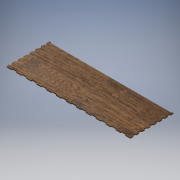
# Autodesk Inventor part: tavolaBase
Saved by Autodesk Inventor 2018.3 (Build 223284000, 284)
## iProperties
Created: 2019-03-04
Part Number: tavolaBase
Material: Generico
Document SubType Name: Modeling
Designer: AlfyPc
Density: 1 g/cm^3
Appearance: Frassino bianco - Giava
Author: AlfyPc
Autodesk Inventor part; units mm, degrees
(part 1 of 2)
ref_plane "YZ Plane" through (0, 0, 0) normal (1, 0, 0) x (0, 1, 0)
ref_plane "XZ Plane" through (0, 0, 0) normal (0, 1, 0) x (-1, 0, 0)
ref_plane "XY Plane" through (0, 0, 0) normal (0, 0, 1) x (1, 0, 0)
sketch "Schizzo1" plane through (0, 0, 0) normal (0, 0, 1) x (1, 0, 0)
  line L0 (233.5, -78.5) -> (-233.5, -78.5)
  line L1 (-233.5, -78.5) -> (-233.5, 78.5)
  line L2 (-233.5, 78.5) -> (233.5, 78.5)
  line L3 (233.5, 78.5) -> (233.5, -78.5)
  line L4 (233.5, -78.5) -> (-233.5, 78.5) construction
  line L5 (-233.5, -78.5) -> (233.5, 78.5) construction
  point P0 (0, 0)
  dimension "d0" = 467
  dimension "d1" = 157
  constraints: 12 end point, 2 midpoint, 2 parallel, 1 horizontal, 1 perpendicular
  measures "d0" distance of L0.start L0.end
  measures "d1" distance of L0.end L1.end
extrude "Estrusione1" add sketch "Schizzo1" against normal blind 4
sketch "Schizzo3" plane through (0, 0, 0) normal (0, 0, 1) x (1, 0, 0)
  line L0 (233.5, -78.5) -> (-233.5, -78.5) projected
  line L1 (233.5, 78.5) -> (233.5, -78.5) projected
  line L2 (-233.5, 78.5) -> (233.5, 78.5) projected
  line L3 (-233.5, -78.5) -> (-233.5, 78.5) projected
  line L4 (-237.5, -82.5) -> (237.5, -82.5) construction
  line L5 (237.5, -82.5) -> (237.5, 82.5) construction
  line L6 (237.5, 82.5) -> (-237.5, 82.5) construction
  line L7 (-237.5, 82.5) -> (-237.5, -82.5) construction
  line L8 (237.5, -82.5) -> (218.5, -82.5)
  line L9 (218.5, -82.5) -> (218.5, -78.5)
  line L10 (218.5, -78.5) -> (237.5, -78.5)
  line L11 (237.5, -78.5) -> (237.5, -82.5)
  line L12 (237.5, 82.5) -> (218.5, 82.5)
  line L13 (218.5, 82.5) -> (218.5, 78.5)
  line L14 (218.5, 78.5) -> (237.5, 78.5)
  line L15 (237.5, 78.5) -> (237.5, 82.5)
  line L16 (237.5, -82.5) -> (233.5, -82.5)
  line L17 (233.5, -82.5) -> (233.5, -71.5)
  line L18 (233.5, -71.5) -> (237.5, -71.5)
  line L19 (237.5, -71.5) -> (237.5, -82.5)
  line L20 (-237.5, -82.5) -> (-233.5, -82.5)
  line L21 (-233.5, -82.5) -> (-233.5, -71.5)
  line L22 (-233.5, -71.5) -> (-237.5, -71.5)
  line L23 (-237.5, -71.5) -> (-237.5, -82.5)
  line L24 (218.5, -78.5) -> (218.5, -82.5)
  line L25 (218.5, -82.5) -> (214.5, -82.5)
  line L26 (199.5, -82.5) -> (199.5, -78.5)
  line L27 (199.5, -78.5) -> (218.5, -78.5)
  line L28 (218.5, -82.5) -> (199.5, -82.5)
  line L29 (199.5, 82.5) -> (199.5, 78.5)
  line L30 (199.5, 78.5) -> (218.5, 78.5)
  line L31 (218.5, 78.5) -> (218.5, 82.5)
  line L32 (218.5, 82.5) -> (199.5, 82.5)
  line L33 (199.5, -78.5) -> (199.5, -82.5)
  line L34 (199.5, -82.5) -> (195.5, -82.5)
  line L35 (180.5, -82.5) -> (180.5, -78.5)
  line L36 (180.5, -78.5) -> (199.5, -78.5)
  line L37 (199.5, -82.5) -> (180.5, -82.5)
  line L38 (180.5, 82.5) -> (180.5, 78.5)
  line L39 (180.5, 78.5) -> (199.5, 78.5)
  line L40 (199.5, 78.5) -> (199.5, 82.5)
  line L41 (199.5, 82.5) -> (180.5, 82.5)
  line L42 (180.5, -78.5) -> (180.5, -82.5)
  line L43 (180.5, -82.5) -> (176.5, -82.5)
  line L44 (161.5, -82.5) -> (161.5, -78.5)
  line L45 (161.5, -78.5) -> (180.5, -78.5)
  line L46 (180.5, -82.5) -> (161.5, -82.5)
  line L47 (161.5, 82.5) -> (161.5, 78.5)
  line L48 (161.5, 78.5) -> (180.5, 78.5)
  line L49 (180.5, 78.5) -> (180.5, 82.5)
  line L50 (180.5, 82.5) -> (161.5, 82.5)
  line L51 (161.5, -78.5) -> (161.5, -82.5)
  line L52 (161.5, -82.5) -> (157.5, -82.5)
  line L53 (142.5, -82.5) -> (142.5, -78.5)
  line L54 (142.5, -78.5) -> (161.5, -78.5)
  line L55 (161.5, -82.5) -> (142.5, -82.5)
  line L56 (142.5, 82.5) -> (142.5, 78.5)
  line L57 (142.5, 78.5) -> (161.5, 78.5)
  line L58 (161.5, 78.5) -> (161.5, 82.5)
  line L59 (161.5, 82.5) -> (142.5, 82.5)
  line L60 (142.5, -78.5) -> (142.5, -82.5)
  line L61 (142.5, -82.5) -> (138.5, -82.5)
  line L62 (123.5, -82.5) -> (123.5, -78.5)
  line L63 (123.5, -78.5) -> (142.5, -78.5)
  line L64 (142.5, -82.5) -> (123.5, -82.5)
  line L65 (123.5, 82.5) -> (123.5, 78.5)
  line L66 (123.5, 78.5) -> (142.5, 78.5)
  line L67 (142.5, 78.5) -> (142.5, 82.5)
  line L68 (142.5, 82.5) -> (123.5, 82.5)
  line L69 (123.5, -78.5) -> (123.5, -82.5)
  line L70 (123.5, -82.5) -> (119.5, -82.5)
  line L71 (104.5, -82.5) -> (104.5, -78.5)
  line L72 (104.5, -78.5) -> (123.5, -78.5)
  line L73 (123.5, -82.5) -> (104.5, -82.5)
  line L74 (104.5, 82.5) -> (104.5, 78.5)
  line L75 (104.5, 78.5) -> (123.5, 78.5)
  line L76 (123.5, 78.5) -> (123.5, 82.5)
  line L77 (123.5, 82.5) -> (104.5, 82.5)
  line L78 (104.5, -78.5) -> (104.5, -82.5)
  line L79 (104.5, -82.5) -> (100.5, -82.5)
  line L80 (85.5, -82.5) -> (85.5, -78.5)
  line L81 (85.5, -78.5) -> (104.5, -78.5)
  line L82 (104.5, -82.5) -> (85.5, -82.5)
  line L83 (85.5, 82.5) -> (85.5, 78.5)
  line L84 (85.5, 78.5) -> (104.5, 78.5)
  line L85 (104.5, 78.5) -> (104.5, 82.5)
  line L86 (104.5, 82.5) -> (85.5, 82.5)
  line L87 (85.5, -78.5) -> (85.5, -82.5)
  line L88 (85.5, -82.5) -> (81.5, -82.5)
  line L89 (66.5, -82.5) -> (66.5, -78.5)
  line L90 (66.5, -78.5) -> (85.5, -78.5)
  line L91 (85.5, -82.5) -> (66.5, -82.5)
  line L92 (66.5, 82.5) -> (66.5, 78.5)
  line L93 (66.5, 78.5) -> (85.5, 78.5)
  line L94 (85.5, 78.5) -> (85.5, 82.5)
  line L95 (85.5, 82.5) -> (66.5, 82.5)
  line L96 (66.5, -78.5) -> (66.5, -82.5)
  line L97 (66.5, -82.5) -> (62.5, -82.5)
  line L98 (47.5, -82.5) -> (47.5, -78.5)
  line L99 (47.5, -78.5) -> (66.5, -78.5)
  line L100 (66.5, -82.5) -> (47.5, -82.5)
  line L101 (47.5, 82.5) -> (47.5, 78.5)
  line L102 (47.5, 78.5) -> (66.5, 78.5)
  line L103 (66.5, 78.5) -> (66.5, 82.5)
  line L104 (66.5, 82.5) -> (47.5, 82.5)
  line L105 (47.5, -78.5) -> (47.5, -82.5)
  line L106 (47.5, -82.5) -> (43.5, -82.5)
  line L107 (28.5, -82.5) -> (28.5, -78.5)
  line L108 (28.5, -78.5) -> (47.5, -78.5)
  line L109 (47.5, -82.5) -> (28.5, -82.5)
  line L110 (28.5, 82.5) -> (28.5, 78.5)
  line L111 (28.5, 78.5) -> (47.5, 78.5)
  line L112 (47.5, 78.5) -> (47.5, 82.5)
  line L113 (47.5, 82.5) -> (28.5, 82.5)
  line L114 (28.5, -78.5) -> (28.5, -82.5)
  line L115 (28.5, -82.5) -> (24.5, -82.5)
  line L116 (9.5, -82.5) -> (9.5, -78.5)
  line L117 (9.5, -78.5) -> (28.5, -78.5)
  line L118 (28.5, -82.5) -> (9.5, -82.5)
  line L119 (9.5, 82.5) -> (9.5, 78.5)
  line L120 (9.5, 78.5) -> (28.5, 78.5)
  line L121 (28.5, 78.5) -> (28.5, 82.5)
  line L122 (28.5, 82.5) -> (9.5, 82.5)
  line L123 (9.5, -78.5) -> (9.5, -82.5)
  line L124 (9.5, -82.5) -> (5.5, -82.5)
  line L125 (-9.5, -82.5) -> (-9.5, -78.5)
  line L126 (-9.5, -78.5) -> (9.5, -78.5)
  line L127 (9.5, -82.5) -> (-9.5, -82.5)
  line L128 (-9.5, 82.5) -> (-9.5, 78.5)
  line L129 (-9.5, 78.5) -> (9.5, 78.5)
  line L130 (9.5, 78.5) -> (9.5, 82.5)
  line L131 (9.5, 82.5) -> (-9.5, 82.5)
  line L132 (-9.5, -78.5) -> (-9.5, -82.5)
  line L133 (-9.5, -82.5) -> (-13.5, -82.5)
  line L134 (-28.5, -82.5) -> (-28.5, -78.5)
  line L135 (-28.5, -78.5) -> (-9.5, -78.5)
  line L136 (-9.5, -82.5) -> (-28.5, -82.5)
  line L137 (-28.5, 82.5) -> (-28.5, 78.5)
  line L138 (-28.5, 78.5) -> (-9.5, 78.5)
  line L139 (-9.5, 78.5) -> (-9.5, 82.5)
  line L140 (-9.5, 82.5) -> (-28.5, 82.5)
  line L141 (-28.5, -78.5) -> (-28.5, -82.5)
  line L142 (-28.5, -82.5) -> (-32.5, -82.5)
  line L143 (-47.5, -82.5) -> (-47.5, -78.5)
  line L144 (-47.5, -78.5) -> (-28.5, -78.5)
  line L145 (-28.5, -82.5) -> (-47.5, -82.5)
  line L146 (-47.5, 82.5) -> (-47.5, 78.5)
  line L147 (-47.5, 78.5) -> (-28.5, 78.5)
  line L148 (-28.5, 78.5) -> (-28.5, 82.5)
  line L149 (-28.5, 82.5) -> (-47.5, 82.5)
  line L150 (-47.5, -78.5) -> (-47.5, -82.5)
  line L151 (-47.5, -82.5) -> (-51.5, -82.5)
  line L152 (-66.5, -82.5) -> (-66.5, -78.5)
  line L153 (-66.5, -78.5) -> (-47.5, -78.5)
  line L154 (-47.5, -82.5) -> (-66.5, -82.5)
  line L155 (-66.5, 82.5) -> (-66.5, 78.5)
  line L156 (-66.5, 78.5) -> (-47.5, 78.5)
  line L157 (-47.5, 78.5) -> (-47.5, 82.5)
  line L158 (-47.5, 82.5) -> (-66.5, 82.5)
  line L159 (-66.5, -78.5) -> (-66.5, -82.5)
  line L160 (-66.5, -82.5) -> (-70.5, -82.5)
  line L161 (-85.5, -82.5) -> (-85.5, -78.5)
  line L162 (-85.5, -78.5) -> (-66.5, -78.5)
  line L163 (-66.5, -82.5) -> (-85.5, -82.5)
  line L164 (-85.5, 82.5) -> (-85.5, 78.5)
  line L165 (-85.5, 78.5) -> (-66.5, 78.5)
  line L166 (-66.5, 78.5) -> (-66.5, 82.5)
  line L167 (-66.5, 82.5) -> (-85.5, 82.5)
  line L168 (-85.5, -78.5) -> (-85.5, -82.5)
  line L169 (-85.5, -82.5) -> (-89.5, -82.5)
  line L170 (-104.5, -82.5) -> (-104.5, -78.5)
  line L171 (-104.5, -78.5) -> (-85.5, -78.5)
  line L172 (-85.5, -82.5) -> (-104.5, -82.5)
  line L173 (-104.5, 82.5) -> (-104.5, 78.5)
  line L174 (-104.5, 78.5) -> (-85.5, 78.5)
  line L175 (-85.5, 78.5) -> (-85.5, 82.5)
  line L176 (-85.5, 82.5) -> (-104.5, 82.5)
  line L177 (-104.5, -78.5) -> (-104.5, -82.5)
  line L178 (-104.5, -82.5) -> (-108.5, -82.5)
  line L179 (-123.5, -82.5) -> (-123.5, -78.5)
  line L180 (-123.5, -78.5) -> (-104.5, -78.5)
  line L181 (-104.5, -82.5) -> (-123.5, -82.5)
  line L182 (-123.5, 82.5) -> (-123.5, 78.5)
  line L183 (-123.5, 78.5) -> (-104.5, 78.5)
  line L184 (-104.5, 78.5) -> (-104.5, 82.5)
  line L185 (-104.5, 82.5) -> (-123.5, 82.5)
  line L186 (-123.5, -78.5) -> (-123.5, -82.5)
  line L187 (-123.5, -82.5) -> (-127.5, -82.5)
  line L188 (-142.5, -82.5) -> (-142.5, -78.5)
  line L189 (-142.5, -78.5) -> (-123.5, -78.5)
  line L190 (-123.5, -82.5) -> (-142.5, -82.5)
  line L191 (-142.5, 82.5) -> (-142.5, 78.5)
  line L192 (-142.5, 78.5) -> (-123.5, 78.5)
  line L193 (-123.5, 78.5) -> (-123.5, 82.5)
  line L194 (-123.5, 82.5) -> (-142.5, 82.5)
  line L195 (-142.5, -78.5) -> (-142.5, -82.5)
  line L196 (-142.5, -82.5) -> (-146.5, -82.5)
  line L197 (-161.5, -82.5) -> (-161.5, -78.5)
  line L198 (-161.5, -78.5) -> (-142.5, -78.5)
  line L199 (-142.5, -82.5) -> (-161.5, -82.5)
  line L200 (-161.5, 82.5) -> (-161.5, 78.5)
  line L201 (-161.5, 78.5) -> (-142.5, 78.5)
  line L202 (-142.5, 78.5) -> (-142.5, 82.5)
  line L203 (-142.5, 82.5) -> (-161.5, 82.5)
  line L204 (-161.5, -78.5) -> (-161.5, -82.5)
  line L205 (-161.5, -82.5) -> (-165.5, -82.5)
  line L206 (-180.5, -82.5) -> (-180.5, -78.5)
  line L207 (-180.5, -78.5) -> (-161.5, -78.5)
  line L208 (-161.5, -82.5) -> (-180.5, -82.5)
  line L209 (-180.5, 82.5) -> (-180.5, 78.5)
  line L210 (-180.5, 78.5) -> (-161.5, 78.5)
  line L211 (-161.5, 78.5) -> (-161.5, 82.5)
  line L212 (-161.5, 82.5) -> (-180.5, 82.5)
  line L213 (-180.5, -78.5) -> (-180.5, -82.5)
  line L214 (-180.5, -82.5) -> (-184.5, -82.5)
  line L215 (-199.5, -82.5) -> (-199.5, -78.5)
  line L216 (-199.5, -78.5) -> (-180.5, -78.5)
  line L217 (-180.5, -82.5) -> (-199.5, -82.5)
  line L218 (-199.5, 82.5) -> (-199.5, 78.5)
  line L219 (-199.5, 78.5) -> (-180.5, 78.5)
  line L220 (-180.5, 78.5) -> (-180.5, 82.5)
  line L221 (-180.5, 82.5) -> (-199.5, 82.5)
  line L222 (-199.5, -78.5) -> (-199.5, -82.5)
  line L223 (-199.5, -82.5) -> (-203.5, -82.5)
  line L224 (-218.5, -82.5) -> (-218.5, -78.5)
  line L225 (-218.5, -78.5) -> (-199.5, -78.5)
  line L226 (-199.5, -82.5) -> (-218.5, -82.5)
  line L227 (-218.5, 82.5) -> (-218.5, 78.5)
  line L228 (-218.5, 78.5) -> (-199.5, 78.5)
  line L229 (-199.5, 78.5) -> (-199.5, 82.5)
  line L230 (-199.5, 82.5) -> (-218.5, 82.5)
  line L231 (-218.5, -78.5) -> (-218.5, -82.5)
  line L232 (-218.5, -82.5) -> (-222.5, -82.5)
  line L233 (-237.5, -82.5) -> (-237.5, -78.5)
  line L234 (-237.5, -78.5) -> (-218.5, -78.5)
  line L235 (-218.5, -82.5) -> (-237.5, -82.5)
  line L236 (-237.5, 82.5) -> (-237.5, 78.5)
  line L237 (-237.5, 78.5) -> (-218.5, 78.5)
  line L238 (-218.5, 78.5) -> (-218.5, 82.5)
  line L239 (-218.5, 82.5) -> (-237.5, 82.5)
  line L240 (237.5, -67.5) -> (237.5, -71.5)
  line L241 (237.5, -71.5) -> (233.5, -71.5)
  line L242 (233.5, -60.5) -> (237.5, -60.5)
  line L243 (237.5, -60.5) -> (237.5, -71.5)
  line L244 (233.5, -71.5) -> (233.5, -60.5)
  line L245 (-237.5, -71.5) -> (-233.5, -71.5)
  line L246 (-233.5, -71.5) -> (-233.5, -60.5)
  line L247 (-233.5, -60.5) -> (-237.5, -60.5)
  line L248 (-237.5, -60.5) -> (-237.5, -71.5)
  line L249 (-237.5, -71.5) -> (-237.5, -67.5)
  line L250 (237.5, -56.5) -> (237.5, -60.5)
  line L251 (237.5, -60.5) -> (233.5, -60.5)
  line L252 (233.5, -49.5) -> (237.5, -49.5)
  line L253 (237.5, -49.5) -> (237.5, -60.5)
  line L254 (233.5, -60.5) -> (233.5, -49.5)
  line L255 (-237.5, -60.5) -> (-233.5, -60.5)
  line L256 (-233.5, -60.5) -> (-233.5, -49.5)
  line L257 (-233.5, -49.5) -> (-237.5, -49.5)
  line L258 (-237.5, -49.5) -> (-237.5, -60.5)
  line L259 (-237.5, -60.5) -> (-237.5, -56.5)
  line L260 (237.5, -45.5) -> (237.5, -49.5)
  line L261 (237.5, -49.5) -> (233.5, -49.5)
  line L262 (233.5, -38.5) -> (237.5, -38.5)
  line L263 (237.5, -38.5) -> (237.5, -49.5)
  line L264 (233.5, -49.5) -> (233.5, -38.5)
  line L265 (-237.5, -49.5) -> (-233.5, -49.5)
  line L266 (-233.5, -49.5) -> (-233.5, -38.5)
  line L267 (-233.5, -38.5) -> (-237.5, -38.5)
  line L268 (-237.5, -38.5) -> (-237.5, -49.5)
  line L269 (-237.5, -49.5) -> (-237.5, -45.5)
  line L270 (237.5, -34.5) -> (237.5, -38.5)
  line L271 (237.5, -38.5) -> (233.5, -38.5)
  line L272 (233.5, -27.5) -> (237.5, -27.5)
  line L273 (237.5, -27.5) -> (237.5, -38.5)
  line L274 (233.5, -38.5) -> (233.5, -27.5)
  line L275 (-237.5, -38.5) -> (-233.5, -38.5)
  line L276 (-233.5, -38.5) -> (-233.5, -27.5)
  line L277 (-233.5, -27.5) -> (-237.5, -27.5)
  line L278 (-237.5, -27.5) -> (-237.5, -38.5)
  line L279 (-237.5, -38.5) -> (-237.5, -34.5)
  line L280 (237.5, -23.5) -> (237.5, -27.5)
  line L281 (237.5, -27.5) -> (233.5, -27.5)
  line L282 (233.5, -16.5) -> (237.5, -16.5)
  line L283 (237.5, -16.5) -> (237.5, -27.5)
  line L284 (233.5, -27.5) -> (233.5, -16.5)
  line L285 (-237.5, -27.5) -> (-233.5, -27.5)
  line L286 (-233.5, -27.5) -> (-233.5, -16.5)
  line L287 (-233.5, -16.5) -> (-237.5, -16.5)
  line L288 (-237.5, -16.5) -> (-237.5, -27.5)
  line L289 (-237.5, -27.5) -> (-237.5, -23.5)
  line L290 (237.5, -12.5) -> (237.5, -16.5)
  line L291 (237.5, -16.5) -> (233.5, -16.5)
  line L292 (233.5, -5.5) -> (237.5, -5.5)
  line L293 (237.5, -5.5) -> (237.5, -16.5)
  line L294 (233.5, -16.5) -> (233.5, -5.5)
  line L295 (-237.5, -16.5) -> (-233.5, -16.5)
  line L296 (-233.5, -16.5) -> (-233.5, -5.5)
  line L297 (-233.5, -5.5) -> (-237.5, -5.5)
  line L298 (-237.5, -5.5) -> (-237.5, -16.5)
  line L299 (-237.5, -16.5) -> (-237.5, -12.5)
  line L300 (237.5, -1.5) -> (237.5, -5.5)
  line L301 (237.5, -5.5) -> (233.5, -5.5)
  line L302 (233.5, 5.5) -> (237.5, 5.5)
  line L303 (237.5, 5.5) -> (237.5, -5.5)
  line L304 (233.5, -5.5) -> (233.5, 5.5)
  line L305 (-237.5, -5.5) -> (-233.5, -5.5)
  line L306 (-233.5, -5.5) -> (-233.5, 5.5)
  line L307 (-233.5, 5.5) -> (-237.5, 5.5)
  line L308 (-237.5, 5.5) -> (-237.5, -5.5)
  line L309 (-237.5, -5.5) -> (-237.5, -1.5)
  line L310 (237.5, 9.5) -> (237.5, 5.5)
  line L311 (237.5, 5.5) -> (233.5, 5.5)
  line L312 (233.5, 16.5) -> (237.5, 16.5)
  line L313 (237.5, 16.5) -> (237.5, 5.5)
  line L314 (233.5, 5.5) -> (233.5, 16.5)
  line L315 (-237.5, 5.5) -> (-233.5, 5.5)
  line L316 (-233.5, 5.5) -> (-233.5, 16.5)
  line L317 (-233.5, 16.5) -> (-237.5, 16.5)
  line L318 (-237.5, 16.5) -> (-237.5, 5.5)
  line L319 (-237.5, 5.5) -> (-237.5, 9.5)
  line L320 (237.5, 20.5) -> (237.5, 16.5)
  line L321 (237.5, 16.5) -> (233.5, 16.5)
  line L322 (233.5, 27.5) -> (237.5, 27.5)
  line L323 (237.5, 27.5) -> (237.5, 16.5)
  line L324 (233.5, 16.5) -> (233.5, 27.5)
  line L325 (-237.5, 16.5) -> (-233.5, 16.5)
  line L326 (-233.5, 16.5) -> (-233.5, 27.5)
  line L327 (-233.5, 27.5) -> (-237.5, 27.5)
  line L328 (-237.5, 27.5) -> (-237.5, 16.5)
  line L329 (-237.5, 16.5) -> (-237.5, 20.5)
  line L330 (237.5, 31.5) -> (237.5, 27.5)
  line L331 (237.5, 27.5) -> (233.5, 27.5)
  line L332 (233.5, 38.5) -> (237.5, 38.5)
  line L333 (237.5, 38.5) -> (237.5, 27.5)
  line L334 (233.5, 27.5) -> (233.5, 38.5)
  line L335 (-237.5, 27.5) -> (-233.5, 27.5)
  line L336 (-233.5, 27.5) -> (-233.5, 38.5)
  line L337 (-233.5, 38.5) -> (-237.5, 38.5)
  line L338 (-237.5, 38.5) -> (-237.5, 27.5)
  line L339 (-237.5, 27.5) -> (-237.5, 31.5)
  line L340 (237.5, 42.5) -> (237.5, 38.5)
  line L341 (237.5, 38.5) -> (233.5, 38.5)
  line L342 (233.5, 49.5) -> (237.5, 49.5)
  line L343 (237.5, 49.5) -> (237.5, 38.5)
  line L344 (233.5, 38.5) -> (233.5, 49.5)
  line L345 (-237.5, 38.5) -> (-233.5, 38.5)
  line L346 (-233.5, 38.5) -> (-233.5, 49.5)
  line L347 (-233.5, 49.5) -> (-237.5, 49.5)
  line L348 (-237.5, 49.5) -> (-237.5, 38.5)
  line L349 (-237.5, 38.5) -> (-237.5, 42.5)
  line L350 (237.5, 53.5) -> (237.5, 49.5)
  line L351 (237.5, 49.5) -> (233.5, 49.5)
  line L352 (233.5, 60.5) -> (237.5, 60.5)
  line L353 (237.5, 60.5) -> (237.5, 49.5)
  line L354 (233.5, 49.5) -> (233.5, 60.5)
  line L355 (-237.5, 49.5) -> (-233.5, 49.5)
  line L356 (-233.5, 49.5) -> (-233.5, 60.5)
  line L357 (-233.5, 60.5) -> (-237.5, 60.5)
  line L358 (-237.5, 60.5) -> (-237.5, 49.5)
  line L359 (-237.5, 49.5) -> (-237.5, 53.5)
  line L360 (237.5, 64.5) -> (237.5, 60.5)
  line L361 (237.5, 60.5) -> (233.5, 60.5)
  line L362 (233.5, 71.5) -> (237.5, 71.5)
  line L363 (237.5, 71.5) -> (237.5, 60.5)
  line L364 (233.5, 60.5) -> (233.5, 71.5)
  line L365 (-237.5, 60.5) -> (-233.5, 60.5)
  line L366 (-233.5, 60.5) -> (-233.5, 71.5)
  line L367 (-233.5, 71.5) -> (-237.5, 71.5)
  line L368 (-237.5, 71.5) -> (-237.5, 60.5)
  line L369 (-237.5, 60.5) -> (-237.5, 64.5)
  line L370 (237.5, 75.5) -> (237.5, 71.5)
  line L371 (237.5, 71.5) -> (233.5, 71.5)
  line L372 (233.5, 82.5) -> (237.5, 82.5)
  line L373 (237.5, 82.5) -> (237.5, 71.5)
  line L374 (233.5, 71.5) -> (233.5, 82.5)
  line L375 (-237.5, 71.5) -> (-233.5, 71.5)
  line L376 (-233.5, 71.5) -> (-233.5, 82.5)
  line L377 (-233.5, 82.5) -> (-237.5, 82.5)
  line L378 (-237.5, 82.5) -> (-237.5, 71.5)
  line L379 (-237.5, 71.5) -> (-237.5, 75.5)
  point P0 (0, 0)
  point P1 (214.5, -78.5)
  point P2 (214.5, 78.5)
  point P3 (195.5, -78.5)
  point P4 (195.5, 78.5)
  point P5 (176.5, -78.5)
  point P6 (176.5, 78.5)
  point P7 (157.5, -78.5)
  point P8 (157.5, 78.5)
  point P9 (138.5, -78.5)
  point P10 (138.5, 78.5)
  point P11 (119.5, -78.5)
  point P12 (119.5, 78.5)
  point P13 (100.5, -78.5)
  point P14 (100.5, 78.5)
  point P15 (81.5, -78.5)
  point P16 (81.5, 78.5)
  point P17 (62.5, -78.5)
  point P18 (62.5, 78.5)
  point P19 (43.5, -78.5)
  point P20 (43.5, 78.5)
  point P21 (24.5, -78.5)
  point P22 (24.5, 78.5)
  point P23 (5.5, -78.5)
  point P24 (5.5, 78.5)
  point P25 (-13.5, -78.5)
  point P26 (-13.5, 78.5)
  point P27 (-32.5, -78.5)
  point P28 (-32.5, 78.5)
  point P29 (-51.5, -78.5)
  point P30 (-51.5, 78.5)
  point P31 (-70.5, -78.5)
  point P32 (-70.5, 78.5)
  point P33 (-89.5, -78.5)
  point P34 (-89.5, 78.5)
  point P35 (-108.5, -78.5)
  point P36 (-108.5, 78.5)
  point P37 (-127.5, -78.5)
  point P38 (-127.5, 78.5)
  point P39 (-146.5, -78.5)
  point P40 (-146.5, 78.5)
  point P41 (-165.5, -78.5)
  point P42 (-165.5, 78.5)
  point P43 (-184.5, -78.5)
  point P44 (-184.5, 78.5)
  point P45 (-203.5, -78.5)
  point P46 (-203.5, 78.5)
  point P47 (-222.5, -78.5)
  point P48 (-222.5, 78.5)
  point P49 (233.5, -67.5)
  point P50 (-233.5, -67.5)
  point P51 (233.5, -56.5)
  point P52 (-233.5, -56.5)
  point P53 (233.5, -45.5)
  point P54 (-233.5, -45.5)
  point P55 (233.5, -34.5)
  point P56 (-233.5, -34.5)
  point P57 (233.5, -23.5)
  point P58 (-233.5, -23.5)
  point P59 (233.5, -12.5)
  point P60 (-233.5, -12.5)
  point P61 (233.5, -1.5)
  point P62 (-233.5, -1.5)
  point P63 (233.5, 9.5)
  point P64 (-233.5, 9.5)
  point P65 (233.5, 20.5)
  point P66 (-233.5, 20.5)
  point P67 (233.5, 31.5)
  point P68 (-233.5, 31.5)
  point P69 (233.5, 42.5)
  point P70 (-233.5, 42.5)
  point P71 (233.5, 53.5)
  point P72 (-233.5, 53.5)
  point P73 (233.5, 64.5)
  point P74 (-233.5, 64.5)
  point P75 (233.5, 75.5)
  point P76 (-233.5, 75.5)
  dimension "d28" = 4
  dimension "d29" = 475
  dimension "d30" = 165
  dimension "d31" = 19
  dimension "d32" = 4
  dimension "d33" = 19
  dimension "d34" = 4
  dimension "d35" = 4
  dimension "d36" = 11
  dimension "d37" = 4
  dimension "d38" = 11
  dimension "d41" = 19
  dimension "d48" = 11
  constraints: 752 end point, 8 parallel, 5 horizontal, 4 perpendicular, 1 vertical, 805 other
  measures "d28" distance between parallel lines of L0 L4
  measures "d29" distance of L4.start L4.end
  measures "d30" distance of L4.end L5.end
  measures "d31" distance of L9.end L10.end
  measures "d32" distance of L8.end L9.end
  measures "d33" distance of L14.end L13.end
  measures "d34" distance of L13.end L12.end
  measures "d35" distance of L17.end L18.end
  measures "d36" distance of L16.end L17.end
  measures "d37" distance of L22.end L21.end
  measures "d38" distance of L21.end L20.end
  measures "d41" distance of L10.end L24.start
  measures "d48" distance of L0.start point (233.5, -67.5)
extrude "Estrusione2" add sketch "Schizzo3" against normal up to surface (4 mm away) contours L17 L8 L9 L0 | L1 L18 L19 L10 | L10 L11 L8 L17 | L26 L34 L37 L35 L0 | L1 L252 L253 L250 L242 | L44 L52 L55 L53 L0 | L1 L272 L273 L270 L262 | L62 L70 L73 L71 L0 | L1 L292 L293 L290 L282 | L80 L88 L91 L89 L0 | L1 L312 L313 L310 L302 | L98 L106 L109 L107 L0 | L1 L332 L333 L330 L322 | L116 L124 L127 L125 L0 | L1 L352 L353 L350 L342 | L134 L142 L145 L143 L0 | L1 L14 L373 L370 L362 | L374 L12 L15 L14 | L152 L160 L163 L161 L0 | L170 L178 L181 L179 L0 | L188 L196 L199 L197 L0 | L206 L214 L217 L215 L0 | L224 L232 L235 L21 L0 | L234 L23 L22 L3 | L21 L20 L23 L234 | L247 L258 L257 L3 | L267 L278 L277 L3 | L287 L298 L297 L3 | L307 L318 L317 L3 | L327 L338 L337 L3 | L347 L358 L357 L3 | L367 L378 L237 L3 | L237 L236 L239 L376
sketch "Schizzo4" plane through (0, 0, 0) normal (0, 0, 1) x (1, 0, 0)
  circle A0 centre (29.075, -39.395) radius 1.5
  circle A1 centre (29.075, 41.885) radius 1.5
  circle A2 centre (-135.39, -38.76) radius 1.5
  circle A3 centre (-173.97, 42.5) radius 1.375
  circle A4 centre (-222.97, 42.5) radius 1.375
  circle A5 centre (-173.97, -15.5) radius 1.375
  circle A6 centre (-222.97, -15.5) radius 1.375
  point P0 (0, 0)
extrude "Estrusione3" cut sketch "Schizzo4" against normal blind 10
sketch "Schizzo5" plane through (0, 0, 0) normal (0, 0, 1) x (1, 0, 0)
  circle A0 centre (29.075, 41.885) radius 1.5 projected
  circle A1 centre (-222.97, -15.5) radius 1.375 projected
  circle A2 centre (-222.97, 42.5) radius 1.375 projected
  circle A3 centre (-173.97, 42.5) radius 1.375 projected
  circle A4 centre (-173.97, -15.5) radius 1.375 projected
  circle A5 centre (29.075, -39.395) radius 1.5 projected
  circle A6 centre (-135.39, -38.76) radius 1.5 projected
  line L0 (218.5, -82.5) -> (218.5, -78.5) projected
  line L1 (237.5, -82.5) -> (218.5, -82.5) projected
  line L2 (237.5, -71.5) -> (237.5, -82.5) projected
  line L3 (233.5, -71.5) -> (237.5, -71.5) projected
  line L4 (233.5, -60.5) -> (233.5, -71.5) projected
  line L5 (237.5, -60.5) -> (233.5, -60.5) projected
  line L6 (237.5, -49.5) -> (237.5, -60.5) projected
  line L7 (233.5, -49.5) -> (237.5, -49.5) projected
  line L8 (233.5, -38.5) -> (233.5, -49.5) projected
  line L9 (237.5, -38.5) -> (233.5, -38.5) projected
  line L10 (237.5, -27.5) -> (237.5, -38.5) projected
  line L11 (233.5, -27.5) -> (237.5, -27.5) projected
  line L12 (233.5, -16.5) -> (233.5, -27.5) projected
  line L13 (237.5, -16.5) -> (233.5, -16.5) projected
  line L14 (237.5, -5.5) -> (237.5, -16.5) projected
  line L15 (233.5, -5.5) -> (237.5, -5.5) projected
  line L16 (233.5, 5.5) -> (233.5, -5.5) projected
  line L17 (237.5, 5.5) -> (233.5, 5.5) projected
  line L18 (237.5, 16.5) -> (237.5, 5.5) projected
  line L19 (233.5, 16.5) -> (237.5, 16.5) projected
  line L20 (233.5, 27.5) -> (233.5, 16.5) projected
  line L21 (237.5, 27.5) -> (233.5, 27.5) projected
  line L22 (237.5, 38.5) -> (237.5, 27.5) projected
  line L23 (233.5, 38.5) -> (237.5, 38.5) projected
  line L24 (233.5, 49.5) -> (233.5, 38.5) projected
  line L25 (237.5, 49.5) -> (233.5, 49.5) projected
  line L26 (237.5, 60.5) -> (237.5, 49.5) projected
  line L27 (233.5, 60.5) -> (237.5, 60.5) projected
  line L28 (233.5, 71.5) -> (233.5, 60.5) projected
  line L29 (237.5, 71.5) -> (233.5, 71.5) projected
  line L30 (237.5, 82.5) -> (237.5, 71.5) projected
  line L31 (233.5, 82.5) -> (237.5, 82.5) projected
  line L32 (233.5, 78.5) -> (233.5, 82.5) projected
  line L33 (-233.5, 78.5) -> (233.5, 78.5) projected
  line L34 (-233.5, 78.5) -> (-233.5, 82.5) projected
  line L35 (-233.5, 82.5) -> (-237.5, 82.5) projected
  line L36 (-237.5, 82.5) -> (-237.5, 71.5) projected
  line L37 (-237.5, 71.5) -> (-233.5, 71.5) projected
  line L38 (-233.5, 60.5) -> (-233.5, 71.5) projected
  line L39 (-233.5, 60.5) -> (-237.5, 60.5) projected
  line L40 (-237.5, 60.5) -> (-237.5, 49.5) projected
  line L41 (-237.5, 49.5) -> (-233.5, 49.5) projected
  line L42 (-233.5, 38.5) -> (-233.5, 49.5) projected
  line L43 (-233.5, 38.5) -> (-237.5, 38.5) projected
  line L44 (-237.5, 38.5) -> (-237.5, 27.5) projected
  line L45 (-237.5, 27.5) -> (-233.5, 27.5) projected
  line L46 (-233.5, 16.5) -> (-233.5, 27.5) projected
  line L47 (-233.5, 16.5) -> (-237.5, 16.5) projected
  line L48 (-237.5, 16.5) -> (-237.5, 5.5) projected
  line L49 (-237.5, 5.5) -> (-233.5, 5.5) projected
  line L50 (-233.5, -5.5) -> (-233.5, 5.5) projected
  line L51 (-233.5, -5.5) -> (-237.5, -5.5) projected
  line L52 (-237.5, -5.5) -> (-237.5, -16.5) projected
  line L53 (-237.5, -16.5) -> (-233.5, -16.5) projected
  line L54 (-233.5, -27.5) -> (-233.5, -16.5) projected
  line L55 (-233.5, -27.5) -> (-237.5, -27.5) projected
  line L56 (-237.5, -27.5) -> (-237.5, -38.5) projected
  line L57 (-237.5, -38.5) -> (-233.5, -38.5) projected
  line L58 (-233.5, -49.5) -> (-233.5, -38.5) projected
  line L59 (-233.5, -49.5) -> (-237.5, -49.5) projected
  line L60 (-237.5, -49.5) -> (-237.5, -60.5) projected
  line L61 (-237.5, -60.5) -> (-233.5, -60.5) projected
  line L62 (-233.5, -71.5) -> (-233.5, -60.5) projected
  line L63 (-233.5, -71.5) -> (-237.5, -71.5) projected
  line L64 (-237.5, -71.5) -> (-237.5, -82.5) projected
  line L65 (-237.5, -82.5) -> (-218.5, -82.5) projected
  line L66 (-218.5, -82.5) -> (-218.5, -78.5) projected
  line L67 (-199.5, -78.5) -> (-218.5, -78.5) projected
  line L68 (-199.5, -78.5) -> (-199.5, -82.5) projected
  line L69 (-199.5, -82.5) -> (-180.5, -82.5) projected
  line L70 (-180.5, -82.5) -> (-180.5, -78.5) projected
  line L71 (-161.5, -78.5) -> (-180.5, -78.5) projected
  line L72 (-161.5, -78.5) -> (-161.5, -82.5) projected
  line L73 (-161.5, -82.5) -> (-142.5, -82.5) projected
  line L74 (-142.5, -82.5) -> (-142.5, -78.5) projected
  line L75 (-123.5, -78.5) -> (-142.5, -78.5) projected
  line L76 (-123.5, -78.5) -> (-123.5, -82.5) projected
  line L77 (-123.5, -82.5) -> (-104.5, -82.5) projected
  line L78 (-104.5, -82.5) -> (-104.5, -78.5) projected
  line L79 (-85.5, -78.5) -> (-104.5, -78.5) projected
  line L80 (-85.5, -78.5) -> (-85.5, -82.5) projected
  line L81 (-85.5, -82.5) -> (-66.5, -82.5) projected
  line L82 (-66.5, -82.5) -> (-66.5, -78.5) projected
  line L83 (-47.5, -78.5) -> (-66.5, -78.5) projected
  line L84 (-47.5, -78.5) -> (-47.5, -82.5) projected
  line L85 (-47.5, -82.5) -> (-28.5, -82.5) projected
  line L86 (-28.5, -82.5) -> (-28.5, -78.5) projected
  line L87 (-9.5, -78.5) -> (-28.5, -78.5) projected
  line L88 (-9.5, -78.5) -> (-9.5, -82.5) projected
  line L89 (-9.5, -82.5) -> (9.5, -82.5) projected
  line L90 (9.5, -82.5) -> (9.5, -78.5) projected
  line L91 (28.5, -78.5) -> (9.5, -78.5) projected
  line L92 (28.5, -78.5) -> (28.5, -82.5) projected
  line L93 (28.5, -82.5) -> (47.5, -82.5) projected
  line L94 (47.5, -82.5) -> (47.5, -78.5) projected
  line L95 (66.5, -78.5) -> (47.5, -78.5) projected
  line L96 (66.5, -78.5) -> (66.5, -82.5) projected
  line L97 (66.5, -82.5) -> (85.5, -82.5) projected
  line L98 (85.5, -82.5) -> (85.5, -78.5) projected
  line L99 (104.5, -78.5) -> (85.5, -78.5) projected
  line L100 (104.5, -78.5) -> (104.5, -82.5) projected
  line L101 (104.5, -82.5) -> (123.5, -82.5) projected
  line L102 (123.5, -82.5) -> (123.5, -78.5) projected
  line L103 (142.5, -78.5) -> (123.5, -78.5) projected
  line L104 (142.5, -78.5) -> (142.5, -82.5) projected
  line L105 (142.5, -82.5) -> (161.5, -82.5) projected
  line L106 (161.5, -82.5) -> (161.5, -78.5) projected
  line L107 (180.5, -78.5) -> (161.5, -78.5) projected
  line L108 (180.5, -78.5) -> (180.5, -82.5) projected
  line L109 (180.5, -82.5) -> (199.5, -82.5) projected
  line L110 (199.5, -82.5) -> (199.5, -78.5) projected
  line L111 (218.5, -78.5) -> (199.5, -78.5) projected
  line L112 (-233.5, 66) -> (-226.5, 66) construction
  circle A7 centre (-226.5, 66) radius 1.65
  line L113 (-233.5, -71.5) -> (-233.5, -60.5) projected
  line L114 (-233.5, -66) -> (-226.5, -66) construction
  circle A8 centre (-226.5, -66) radius 1.65
  line L115 (-199.5, -78.5) -> (-218.5, -78.5) projected
  line L116 (-209, -78.5) -> (-209, -71.5) construction
  line L117 (-47.5, -78.5) -> (-66.5, -78.5) construction
  line L118 (-57, -78.5) -> (-57, -71.5) construction
  line L119 (218.5, -78.5) -> (199.5, -78.5) construction
  line L120 (209, -78.5) -> (209, -71.5) construction
  line L121 (233.5, -66) -> (226.5, -66) construction
  line L122 (233.5, 71.5) -> (233.5, 60.5) construction
  line L123 (233.5, 66) -> (226.5, 66) construction
  circle A9 centre (226.5, -66) radius 1.65
  circle A10 centre (209, -71.5) radius 1.65
  circle A11 centre (226.5, 66) radius 1.65
  circle A12 centre (-209, -71.5) radius 1.65
  circle A13 centre (-57, -71.5) radius 1.65
  point P0 (0, 0)
  dimension "d57" = 7
  dimension "d58" = 3.3
  dimension "d59" = 7
  dimension "d60" = 3.3
  dimension "d61" = 7
  dimension "d62" = 7
  dimension "d63" = 7
  dimension "d64" = 7
  dimension "d65" = 7
  dimension "d66" = 3.3
  dimension "d67" = 3.3
  dimension "d68" = 3.3
  dimension "d69" = 3.3
  dimension "d70" = 3.3
  constraints: 14 end point, 7 centre point, 7 coincident, 7 midpoint, 4 horizontal, 3 vertical
  measures "d57" distance of L112.start L112.end
  measures "d58" diameter of A7
  measures "d59" distance of L114.start L114.end
  measures "d60" diameter of A8
  measures "d61" distance of L116.start L116.end
  measures "d62" distance of L118.start L118.end
  measures "d63" distance of L120.start L120.end
  measures "d64" distance of L121.start L121.end
  measures "d65" distance of L123.start L123.end
  measures "d66" diameter of A9
  measures "d67" diameter of A10
  measures "d68" diameter of A11
  measures "d69" diameter of A12
  measures "d70" diameter of A13
extrude "Estrusione4" cut sketch "Schizzo5" against normal blind 10 contours A7 | A8 | A9 | A10 | A11 | A12 | A13
sketch "Schizzo6" plane through (0, 0, 0) normal (0, 0, 1) x (1, 0, 0)
  line L0 (52.3665, 51.202) -> (0.1546, 51.202) construction
  line L1 (0.1546, 51.202) -> (0.1546, 72.5596) construction
  line L2 (0.1546, 72.5596) -> (52.3665, 72.5596) construction
  line L3 (52.3665, 72.5596) -> (52.3665, 51.202) construction
  line L4 (79.3091, 22.3413) -> (57.8744, 22.3413)
  line L5 (57.8744, 22.3413) -> (57.8744, 67.1838)
  line L6 (57.8744, 67.1838) -> (79.3091, 67.1838)
  line L7 (79.3091, 67.1838) -> (79.3091, 22.3413)
  spline S0 degree 2 poles (52.1245, 54.4305) (52.074, 53.9199) (52.058, 53.6274) knots 0 0 0 1 1 1
  spline S1 degree 2 poles (52.058, 53.6274) (52.0341, 53.2285) (51.9915, 51.8349) (51.9915, 51.5477) knots 0 0 0 1 2 2 2
  spline S2 degree 2 poles (51.9915, 51.5477) (51.9915, 51.4467) (51.9942, 51.2605) knots 0 0 0 1 1 1
  spline S3 degree 2 poles (51.9942, 51.2605) (51.683, 51.2685) (51.5022, 51.2685) knots 0 0 0 1 1 1
  spline S4 degree 2 poles (51.5022, 51.2685) (51.2495, 51.2685) (50.5767, 51.2472) (50.3347, 51.2472) knots 0 0 0 1 2 2 2
  spline S5 degree 2 poles (50.3347, 51.2472) (50.0448, 51.2472) (49.9198, 51.2632) knots 0 0 0 1 1 1
  spline S6 degree 2 poles (49.9198, 51.2632) (49.7576, 51.2844) (49.5156, 51.3908) (49.4332, 51.4706) knots 0 0 0 1 2 2 2
  spline S7 degree 2 poles (49.4332, 51.4706) (49.3428, 51.561) (49.2922, 51.6913) knots 0 0 0 1 1 1
  spline S8 degree 2 poles (49.2922, 51.6913) (49.2337, 51.8403) (49.2337, 52.0105) knots 0 0 0 1 1 1
  spline S9 degree 2 poles (49.2337, 52.0105) (49.2337, 52.1434) (49.3002, 52.3828) (49.4252, 52.5716) (49.5768, 52.6966) (49.7231, 52.7657) (49.848, 52.8003) knots 0 0 0 1 2 3 4 5 5 5
  spline S10 degree 2 poles (49.848, 52.8003) (49.7231, 52.8216) (49.5768, 52.8748) (49.4066, 52.9944) (49.271, 53.1806) (49.2045, 53.4093) (49.2045, 53.537) knots 0 0 0 1 2 3 4 5 5 5
  spline S11 degree 2 poles (49.2045, 53.537) (49.2045, 53.7151) (49.3215, 54.0263) (49.4252, 54.138) knots 0 0 0 1 2 2 2
  spline S12 degree 2 poles (49.4252, 54.138) (49.513, 54.2337) (49.7975, 54.3667) (49.9464, 54.3933) knots 0 0 0 1 2 2 2
  spline S13 degree 2 poles (49.9464, 54.3933) (50.0661, 54.4119) (50.7044, 54.4305) (51.0634, 54.4305) knots 0 0 0 1 2 2 2
  line L8 (51.0634, 54.4305) -> (51.6751, 54.4279)
  line L9 (51.6751, 54.4279) -> (52.1245, 54.4305)
  line L10 (51.1432, 53.7949) -> (50.6964, 53.7949)
  spline S14 degree 2 poles (50.6964, 53.7949) (50.5209, 53.7949) (50.4358, 53.7736) knots 0 0 0 1 1 1
  spline S15 degree 2 poles (50.4358, 53.7736) (50.3347, 53.747) (50.2283, 53.6646) (50.1645, 53.521) (50.1645, 53.4306) knots 0 0 0 1 2 3 3 3
  spline S16 degree 2 poles (50.1645, 53.4306) (50.1645, 53.3561) (50.215, 53.2391) (50.3188, 53.1593) (50.4677, 53.1248) (50.6246, 53.1248) knots 0 0 0 1 2 3 4 4 4
  line L11 (50.6246, 53.1248) -> (51.1139, 53.1248)
  line L12 (51.1139, 53.1248) -> (51.1432, 53.7949)
  line L13 (51.09, 52.4945) -> (50.7602, 52.4945)
  spline S17 degree 2 poles (50.7602, 52.4945) (50.5953, 52.4945) (50.4597, 52.4785) (50.3294, 52.436) (50.2337, 52.3376) (50.1938, 52.2179) (50.1938, 52.1567) knots 0 0 0 1 2 3 4 5 5 5
  spline S18 degree 2 poles (50.1938, 52.1567) (50.1938, 52.0716) (50.2762, 51.936) (50.457, 51.8722) (50.6432, 51.8722) knots 0 0 0 1 2 3 3 3
  line L14 (50.6432, 51.8722) -> (51.0607, 51.8722)
  line L15 (51.0607, 51.8722) -> (51.09, 52.4945)
  spline S19 degree 2 poles (47.4067, 51.9998) (47.1195, 51.9998) (46.5876, 52.1753) (46.2206, 52.5078) (46.0451, 52.9519) (46.0451, 53.2072) knots 0 0 0 1 2 3 4 4 4
  spline S20 degree 2 poles (46.0451, 53.2072) (46.0451, 53.4572) (46.202, 53.904) (46.5717, 54.2975) (47.1461, 54.4917) (47.4679, 54.4917) knots 0 0 0 1 2 3 4 4 4
  spline S21 degree 2 poles (47.4679, 54.4917) (47.7604, 54.4917) (48.3056, 54.3188) (48.6699, 53.9891) (48.8534, 53.529) (48.8534, 53.2763) knots 0 0 0 1 2 3 4 4 4
  spline S22 degree 2 poles (48.8534, 53.2763) (48.8534, 53.0237) (48.6753, 52.5636) (48.287, 52.1966) (47.7152, 51.9998) (47.4067, 51.9998) knots 0 0 0 1 2 3 4 4 4
  spline S23 degree 2 poles (47.4227, 52.6833) (47.5716, 52.6833) (47.803, 52.8375) (47.9226, 53.1301) (47.9226, 53.3056) knots 0 0 0 1 2 3 3 3
  spline S24 degree 2 poles (47.9226, 53.3056) (47.9226, 53.5609) (47.6673, 53.8321) (47.4732, 53.8321) knots 0 0 0 1 2 2 2
  spline S25 degree 2 poles (47.4732, 53.8321) (47.3269, 53.8321) (47.0956, 53.6779) (46.9759, 53.3721) (46.9759, 53.1992) knots 0 0 0 1 2 3 3 3
  spline S26 degree 2 poles (46.9759, 53.1992) (46.9759, 53.0556) (47.069, 52.8216) (47.2817, 52.6833) (47.4227, 52.6833) knots 0 0 0 1 2 3 3 3
  spline S27 degree 2 poles (45.484, 52.7365) (45.4388, 52.5051) (45.4175, 52.3323) (45.3909, 52.1461) knots 0 0 0 1 2 2 2
  spline S28 degree 2 poles (45.3909, 52.1461) (44.7234, 51.9998) (44.242, 51.9998) knots 0 0 0 1 1 1
  spline S29 degree 2 poles (44.242, 51.9998) (43.9681, 51.9998) (43.5134, 52.1222) (43.2581, 52.3961) (43.2581, 52.6514) knots 0 0 0 1 2 3 3 3
  spline S30 degree 2 poles (43.2581, 52.6514) (43.2581, 52.7817) (43.3272, 53.6912) (43.3458, 54.4305) knots 0 0 0 1 2 2 2
  spline S31 degree 2 poles (43.3458, 54.4305) (43.5719, 54.4252) (43.7979, 54.4252) knots 0 0 0 1 1 1
  spline S32 degree 2 poles (43.7979, 54.4252) (44.016, 54.4252) (44.2633, 54.4305) knots 0 0 0 1 1 1
  spline S33 degree 2 poles (44.2633, 54.4305) (44.2314, 54.1752) (44.1915, 53.3774) knots 0 0 0 1 1 1
  spline S34 degree 2 poles (44.1915, 53.3774) (44.2793, 53.4199) (44.3803, 53.4572) (44.6303, 53.5316) (44.7713, 53.5822) (44.875, 53.6619) (44.9202, 53.7444) (44.9202, 53.7949) knots 0 0 0 1 2 3 4 5 6 6 6
  spline S35 degree 2 poles (44.9202, 53.7949) (44.9202, 53.8747) (44.7952, 53.9864) (44.6596, 53.9864) knots 0 0 0 1 2 2 2
  spline S36 degree 2 poles (44.6596, 53.9864) (44.609, 53.9864) (44.5, 53.9704) (44.4016, 53.9385) knots 0 0 0 1 2 2 2
  spline S37 degree 2 poles (44.4016, 53.9385) (44.4681, 54.1167) (44.5612, 54.4598) knots 0 0 0 1 1 1
  spline S38 degree 2 poles (44.5612, 54.4598) (44.7606, 54.4917) (44.9388, 54.4917) knots 0 0 0 1 1 1
  spline S39 degree 2 poles (44.9388, 54.4917) (45.226, 54.4917) (45.609, 54.3321) (45.8164, 53.9731) (45.8164, 53.7949) knots 0 0 0 1 2 3 3 3
  spline S40 degree 2 poles (45.8164, 53.7949) (45.8164, 53.6859) (45.7393, 53.4758) (45.5771, 53.2763) (45.359, 53.1354) (44.9814, 53.0104) (44.6915, 52.9545) knots 0 0 0 1 2 3 4 5 5 5
  spline S41 degree 2 poles (44.6915, 52.9545) (44.5691, 52.9306) (44.367, 52.8774) (44.2819, 52.8375) (44.2287, 52.7843) (44.2048, 52.7258) (44.2048, 52.6939) knots 0 0 0 1 2 3 4 5 5 5
  spline S42 degree 2 poles (44.2048, 52.6939) (44.2048, 52.6062) (44.3537, 52.5104) (44.4973, 52.5104) knots 0 0 0 1 2 2 2
  spline S43 degree 2 poles (44.4973, 52.5104) (44.8963, 52.5104) (45.484, 52.7365) knots 0 0 0 1 1 1
  line L16 (42.8246, 54.4305) -> (42.7528, 53.4013)
  line L17 (42.7528, 53.4013) -> (42.7288, 52.8083)
  spline S44 degree 2 poles (42.7288, 52.8083) (42.7262, 52.6487) (42.7262, 52.4812) knots 0 0 0 1 1 1
  spline S45 degree 2 poles (42.7262, 52.4812) (42.7262, 52.311) (42.7315, 52.061) knots 0 0 0 1 1 1
  spline S46 degree 2 poles (42.7315, 52.061) (42.4523, 52.0663) (42.2874, 52.0663) knots 0 0 0 1 1 1
  spline S47 degree 2 poles (42.2874, 52.0663) (42.0932, 52.0663) (41.8433, 52.061) knots 0 0 0 1 1 1
  line L18 (41.8433, 52.061) -> (41.8539, 52.3216)
  spline S48 degree 2 poles (41.8539, 52.3216) (41.7635, 52.2206) (41.6465, 52.1195) (41.4975, 52.0397) (41.3327, 51.9998) (41.2449, 51.9998) knots 0 0 0 1 2 3 4 4 4
  spline S49 degree 2 poles (41.2449, 51.9998) (41.1625, 51.9998) (41.0587, 52.0238) knots 0 0 0 1 1 1
  spline S50 degree 2 poles (41.0587, 52.0238) (41.0561, 52.2764) (41.0481, 52.4413) knots 0 0 0 1 1 1
  line L19 (41.0481, 52.4413) -> (41.0321, 52.7976)
  spline S51 degree 2 poles (41.0321, 52.7976) (41.1598, 52.7604) (41.2715, 52.7604) knots 0 0 0 1 1 1
  spline S52 degree 2 poles (41.2715, 52.7604) (41.4098, 52.7604) (41.6119, 52.8429) (41.7661, 53.0077) (41.8592, 53.2524) (41.8965, 53.7869) (41.8965, 54.13) knots 0 0 0 1 2 3 4 5 5 5
  spline S53 degree 2 poles (41.8965, 54.13) (41.8965, 54.2523) (41.8885, 54.4305) knots 0 0 0 1 1 1
  spline S54 degree 2 poles (41.8885, 54.4305) (42.1145, 54.4252) (42.3406, 54.4252) knots 0 0 0 1 1 1
  spline S55 degree 2 poles (42.3406, 54.4252) (42.5666, 54.4252) (42.8246, 54.4305) knots 0 0 0 1 1 1
  spline S56 degree 2 poles (38.1653, 54.4305) (38.4126, 54.4252) (38.5775, 54.4252) knots 0 0 0 1 1 1
  spline S57 degree 2 poles (38.5775, 54.4252) (38.7637, 54.4252) (39.0296, 54.4305) knots 0 0 0 1 1 1
  line L20 (39.0296, 54.4305) -> (39.0163, 54.1353)
  spline S58 degree 2 poles (39.0163, 54.1353) (39.1067, 54.2257) (39.2397, 54.3348) (39.4525, 54.4358) (39.6971, 54.4917) (39.8274, 54.4917) knots 0 0 0 1 2 3 4 4 4
  spline S59 degree 2 poles (39.8274, 54.4917) (40.0482, 54.4917) (40.4364, 54.3295) (40.7104, 54.0289) (40.846, 53.6194) (40.846, 53.3987) knots 0 0 0 1 2 3 4 4 4
  spline S60 degree 2 poles (40.846, 53.3987) (40.846, 53.0849) (40.5987, 52.4865) (40.2024, 52.1408) (39.7025, 51.9998) (39.4126, 51.9998) knots 0 0 0 1 2 3 4 4 4
  spline S61 degree 2 poles (39.4126, 51.9998) (39.2184, 51.9998) (38.9605, 52.0344) knots 0 0 0 1 1 1
  spline S62 degree 2 poles (38.9605, 52.0344) (38.9419, 51.7578) (38.9339, 51.2605) knots 0 0 0 1 1 1
  spline S63 degree 2 poles (38.9339, 51.2605) (38.6493, 51.2658) (38.4685, 51.2658) knots 0 0 0 1 1 1
  spline S64 degree 2 poles (38.4685, 51.2658) (38.2345, 51.2658) (37.9951, 51.2605) knots 0 0 0 1 1 1
  spline S65 degree 2 poles (37.9951, 51.2605) (38.0616, 51.9493) (38.1653, 53.9385) (38.1653, 54.4305) knots 0 0 0 1 2 2 2
  spline S66 degree 2 poles (38.9924, 52.6381) (39.1147, 52.6115) (39.2264, 52.6115) knots 0 0 0 1 1 1
  spline S67 degree 2 poles (39.2264, 52.6115) (39.4525, 52.6115) (39.7689, 52.7843) (39.9391, 53.154) (39.9391, 53.3322) knots 0 0 0 1 2 3 3 3
  spline S68 degree 2 poles (39.9391, 53.3322) (39.9391, 53.4678) (39.8434, 53.6832) (39.6439, 53.8082) (39.5243, 53.8082) knots 0 0 0 1 2 3 3 3
  spline S69 degree 2 poles (39.5243, 53.8082) (39.3966, 53.8082) (39.1839, 53.6646) (39.0509, 53.3854) (39.0004, 53.0024) (38.9924, 52.6381) knots 0 0 0 1 2 3 4 4 4
  spline S70 degree 2 poles (34.1337, 52.7471) (33.897, 52.7551) (33.7241, 52.7551) knots 0 0 0 1 1 1
  spline S71 degree 2 poles (33.7241, 52.7551) (33.5459, 52.7551) (33.3305, 52.7471) knots 0 0 0 1 1 1
  spline S72 degree 2 poles (33.3305, 52.7471) (33.3305, 52.8827) (33.3492, 53.0822) (33.3997, 53.3242) (33.4795, 53.5449) (33.5539, 53.7072) (33.6178, 53.8189) knots 0 0 0 1 2 3 4 5 5 5
  spline S73 degree 2 poles (33.6178, 53.8189) (33.4715, 54.0024) (33.2002, 54.3002) (33.0992, 54.4305) knots 0 0 0 1 2 2 2
  spline S74 degree 2 poles (33.0992, 54.4305) (33.4289, 54.4252) (33.6284, 54.4252) knots 0 0 0 1 1 1
  spline S75 degree 2 poles (33.6284, 54.4252) (33.8943, 54.4252) (34.1337, 54.4305) knots 0 0 0 1 1 1
  line L21 (34.1337, 54.4305) -> (34.3172, 54.2018)
  spline S76 degree 2 poles (34.3172, 54.2018) (34.4315, 54.2763) (34.5911, 54.364) (34.8278, 54.4465) (35.0964, 54.4917) (35.2373, 54.4917) knots 0 0 0 1 2 3 4 4 4
  spline S77 degree 2 poles (35.2373, 54.4917) (35.5937, 54.4917) (36.1814, 54.2523) (36.4819, 53.763) (36.4819, 53.4838) knots 0 0 0 1 2 3 3 3
  spline S78 degree 2 poles (36.4819, 53.4838) (36.4819, 53.1673) (36.1149, 52.6647) (35.6522, 52.436) knots 0 0 0 1 2 2 2
  spline S79 degree 2 poles (35.6522, 52.436) (35.7426, 52.287) (35.8091, 52.061) (35.8091, 51.9599) knots 0 0 0 1 2 2 2
  spline S80 degree 2 poles (35.8091, 51.9599) (35.8091, 51.7977) (35.6469, 51.4919) (35.3357, 51.2738) (35.006, 51.202) (34.7932, 51.202) knots 0 0 0 1 2 3 4 4 4
  spline S81 degree 2 poles (34.7932, 51.202) (34.4235, 51.202) (34.0167, 51.2898) knots 0 0 0 1 1 1
  line L22 (34.0167, 51.2898) -> (34.0034, 51.9121)
  line L23 (34.0034, 51.9121) -> (34.0007, 52.0105)
  spline S82 degree 2 poles (34.0007, 52.0105) (34.1629, 51.9413) (34.3783, 51.8934) (34.4714, 51.8934) knots 0 0 0 1 2 2 2
  spline S83 degree 2 poles (34.4714, 51.8934) (34.5858, 51.8934) (34.7586, 51.9573) (34.8464, 52.0849) (34.8464, 52.1541) knots 0 0 0 1 2 3 3 3
  spline S84 degree 2 poles (34.8464, 52.1541) (34.8464, 52.194) (34.8198, 52.287) (34.74, 52.4493) (34.5805, 52.678) (34.4714, 52.8109) (34.3624, 52.9333) knots 0 0 0 1 2 3 4 5 5 5
  line L24 (34.3624, 52.9333) -> (34.1789, 53.1487)
  spline S85 degree 2 poles (34.1789, 53.1487) (34.1629, 53.0955) (34.1496, 53.0264) (34.1363, 52.8562) (34.1337, 52.7471) knots 0 0 0 1 2 3 3 3
  spline S86 degree 2 poles (34.748, 53.6593) (34.8358, 53.5476) (35.1097, 53.2338) (35.2586, 53.0476) knots 0 0 0 1 2 2 2
  spline S87 degree 2 poles (35.2586, 53.0476) (35.3357, 53.0955) (35.4208, 53.1567) (35.49, 53.2231) (35.5485, 53.3215) (35.5751, 53.4173) (35.5751, 53.4678) knots 0 0 0 1 2 3 4 5 5 5
  spline S88 degree 2 poles (35.5751, 53.4678) (35.5751, 53.5715) (35.4607, 53.7417) (35.2639, 53.8268) (35.1469, 53.8268) knots 0 0 0 1 2 3 3 3
  spline S89 degree 2 poles (35.1469, 53.8268) (35.0591, 53.8268) (34.9209, 53.7843) (34.8225, 53.7231) (34.748, 53.6593) knots 0 0 0 1 2 3 3 3
  spline S90 degree 2 poles (28.8441, 53.6566) (28.8707, 53.7923) (28.9505, 54.2816) (28.9638, 54.4172) knots 0 0 0 1 2 2 2
  spline S91 degree 2 poles (28.9638, 54.4172) (29.4611, 54.4917) (29.852, 54.4917) knots 0 0 0 1 1 1
  spline S92 degree 2 poles (29.852, 54.4917) (30.227, 54.4917) (30.8759, 54.3029) (31.4184, 53.8747) (31.6498, 53.295) (31.6498, 52.9333) knots 0 0 0 1 2 3 4 4 4
  spline S93 degree 2 poles (31.6498, 52.9333) (31.6498, 52.5131) (31.336, 51.8429) (30.7483, 51.3935) (30.0462, 51.202) (29.6739, 51.202) knots 0 0 0 1 2 3 4 4 4
  spline S94 degree 2 poles (29.6739, 51.202) (29.3281, 51.202) (28.8229, 51.2898) knots 0 0 0 1 1 1
  line L25 (28.8229, 51.2898) -> (28.8175, 51.4839)
  spline S95 degree 2 poles (28.8175, 51.4839) (28.8149, 51.6142) (28.8042, 51.7658) knots 0 0 0 1 1 1
  line L26 (28.8042, 51.7658) -> (28.7883, 52.0317)
  spline S96 degree 2 poles (28.7883, 52.0317) (29.0595, 51.9653) (29.3973, 51.92) (29.5409, 51.92) knots 0 0 0 1 2 2 2
  spline S97 degree 2 poles (29.5409, 51.92) (29.8547, 51.92) (30.3573, 52.17) (30.6445, 52.6487) (30.6445, 52.9386) knots 0 0 0 1 2 3 3 3
  spline S98 degree 2 poles (30.6445, 52.9386) (30.6445, 53.2019) (30.4025, 53.5795) (29.993, 53.7869) (29.6898, 53.7869) knots 0 0 0 1 2 3 3 3
  spline S99 degree 2 poles (29.6898, 53.7869) (29.5249, 53.7869) (29.1367, 53.7338) (28.8441, 53.6566) knots 0 0 0 1 2 2 2
  spline S100 degree 2 poles (28.2112, 52.7365) (28.166, 52.5051) (28.1447, 52.3323) (28.1181, 52.1461) knots 0 0 0 1 2 2 2
  spline S101 degree 2 poles (28.1181, 52.1461) (27.4506, 51.9998) (26.9693, 51.9998) knots 0 0 0 1 1 1
  spline S102 degree 2 poles (26.9693, 51.9998) (26.6953, 51.9998) (26.2406, 52.1222) (25.9853, 52.3961) (25.9853, 52.6514) knots 0 0 0 1 2 3 3 3
  spline S103 degree 2 poles (25.9853, 52.6514) (25.9853, 52.7817) (26.0544, 53.6912) (26.073, 54.4305) knots 0 0 0 1 2 2 2
  spline S104 degree 2 poles (26.073, 54.4305) (26.2991, 54.4252) (26.5251, 54.4252) knots 0 0 0 1 1 1
  spline S105 degree 2 poles (26.5251, 54.4252) (26.7432, 54.4252) (26.9905, 54.4305) knots 0 0 0 1 1 1
  spline S106 degree 2 poles (26.9905, 54.4305) (26.9586, 54.1752) (26.9187, 53.3774) knots 0 0 0 1 1 1
  spline S107 degree 2 poles (26.9187, 53.3774) (27.0065, 53.4199) (27.1076, 53.4572) (27.3575, 53.5316) (27.4985, 53.5822) (27.6022, 53.6619) (27.6474, 53.7444) (27.6474, 53.7949) knots 0 0 0 1 2 3 4 5 6 6 6
  spline S108 degree 2 poles (27.6474, 53.7949) (27.6474, 53.8747) (27.5224, 53.9864) (27.3868, 53.9864) knots 0 0 0 1 2 2 2
  spline S109 degree 2 poles (27.3868, 53.9864) (27.3363, 53.9864) (27.2272, 53.9704) (27.1288, 53.9385) knots 0 0 0 1 2 2 2
  spline S110 degree 2 poles (27.1288, 53.9385) (27.1953, 54.1167) (27.2884, 54.4598) knots 0 0 0 1 1 1
  spline S111 degree 2 poles (27.2884, 54.4598) (27.4878, 54.4917) (27.666, 54.4917) knots 0 0 0 1 1 1
  spline S112 degree 2 poles (27.666, 54.4917) (27.9532, 54.4917) (28.3362, 54.3321) (28.5436, 53.9731) (28.5436, 53.7949) knots 0 0 0 1 2 3 3 3
  spline S113 degree 2 poles (28.5436, 53.7949) (28.5436, 53.6859) (28.4665, 53.4758) (28.3043, 53.2763) (28.0862, 53.1354) (27.7086, 53.0104) (27.4187, 52.9545) knots 0 0 0 1 2 3 4 5 5 5
  spline S114 degree 2 poles (27.4187, 52.9545) (27.2964, 52.9306) (27.0943, 52.8774) (27.0092, 52.8375) (26.956, 52.7843) (26.932, 52.7258) (26.932, 52.6939) knots 0 0 0 1 2 3 4 5 5 5
  spline S115 degree 2 poles (26.932, 52.6939) (26.932, 52.6062) (27.081, 52.5104) (27.2246, 52.5104) knots 0 0 0 1 2 2 2
  spline S116 degree 2 poles (27.2246, 52.5104) (27.6235, 52.5104) (28.2112, 52.7365) knots 0 0 0 1 1 1
  spline S117 degree 2 poles (25.5678, 54.388) (25.5757, 54.2869) (25.5944, 54.0609) (25.6156, 53.8641) knots 0 0 0 1 2 2 2
  line L27 (25.6156, 53.8641) -> (25.6342, 53.6965)
  spline S118 degree 2 poles (25.6342, 53.6965) (25.4109, 53.7843) (25.0864, 53.8694) (24.9508, 53.8694) knots 0 0 0 1 2 2 2
  spline S119 degree 2 poles (24.9508, 53.8694) (24.8364, 53.8694) (24.6955, 53.8268) (24.6317, 53.7497) (24.6317, 53.7072) knots 0 0 0 1 2 3 3 3
  spline S120 degree 2 poles (24.6317, 53.7072) (24.6317, 53.6699) (24.6795, 53.5981) (24.7646, 53.5343) knots 0 0 0 1 2 2 2
  spline S121 degree 2 poles (24.7646, 53.5343) (24.9534, 53.396) (25.2433, 53.1673) (25.3869, 52.9918) (25.464, 52.787) (25.464, 52.678) knots 0 0 0 1 2 3 4 4 4
  spline S122 degree 2 poles (25.464, 52.678) (25.464, 52.4838) (25.2433, 52.1514) (24.8152, 51.9998) (24.5067, 51.9998) knots 0 0 0 1 2 3 3 3
  spline S123 degree 2 poles (24.5067, 51.9998) (24.1849, 51.9998) (23.6849, 52.0823) knots 0 0 0 1 1 1
  line L28 (23.6849, 52.0823) -> (23.6477, 52.7338)
  spline S124 degree 2 poles (23.6477, 52.7338) (23.9269, 52.6221) (24.1875, 52.6221) knots 0 0 0 1 1 1
  spline S125 degree 2 poles (24.1875, 52.6221) (24.3684, 52.6221) (24.5333, 52.6966) (24.5333, 52.7764) knots 0 0 0 1 2 2 2
  spline S126 degree 2 poles (24.5333, 52.7764) (24.5333, 52.8003) (24.5146, 52.8482) (24.4668, 52.8987) (24.395, 52.9519) (24.1157, 53.146) (24.0386, 53.2099) knots 0 0 0 1 2 3 4 5 5 5
  spline S127 degree 2 poles (24.0386, 53.2099) (23.9083, 53.3109) (23.7727, 53.4864) (23.7009, 53.6832) (23.7009, 53.7923) knots 0 0 0 1 2 3 3 3
  spline S128 degree 2 poles (23.7009, 53.7923) (23.7009, 53.9571) (23.8604, 54.2337) (24.1822, 54.4199) (24.5598, 54.4917) (24.7593, 54.4917) knots 0 0 0 1 2 3 4 4 4
  spline S129 degree 2 poles (24.7593, 54.4917) (24.8923, 54.4917) (25.2992, 54.4465) (25.5678, 54.388) knots 0 0 0 1 2 2 2
  spline S130 degree 2 poles (20.9564, 53.7311) (20.9856, 53.8694) (21.0734, 54.4039) knots 0 0 0 1 1 1
  spline S131 degree 2 poles (21.0734, 54.4039) (21.342, 54.4571) (21.709, 54.4917) (21.8978, 54.4917) knots 0 0 0 1 2 2 2
  spline S132 degree 2 poles (21.8978, 54.4917) (22.1744, 54.4917) (22.6371, 54.4146) (22.9748, 54.2204) (23.2009, 53.9305) (23.3206, 53.5316) (23.3206, 53.3189) knots 0 0 0 1 2 3 4 5 5 5
  spline S133 degree 2 poles (23.3206, 53.3189) (23.3206, 53.0237) (23.0839, 52.4546) (22.7089, 52.1355) (22.2222, 51.9998) (21.9669, 51.9998) knots 0 0 0 1 2 3 4 4 4
  spline S134 degree 2 poles (21.9669, 51.9998) (21.7037, 51.9998) (21.2223, 52.1222) (20.8872, 52.428) (20.7463, 52.8136) (20.7463, 53.037) knots 0 0 0 1 2 3 4 4 4
  spline S135 degree 2 poles (20.7463, 53.037) (20.7463, 53.17) (20.7755, 53.3322) knots 0 0 0 1 1 1
  line L29 (20.7755, 53.3322) -> (22.4031, 53.3348)
  spline S136 degree 2 poles (22.4031, 53.3348) (22.4057, 53.3721) (22.4057, 53.4013) knots 0 0 0 1 1 1
  spline S137 degree 2 poles (22.4057, 53.4013) (22.4057, 53.6513) (22.0467, 53.888) (21.7914, 53.888) knots 0 0 0 1 2 2 2
  spline S138 degree 2 poles (21.7914, 53.888) (21.6372, 53.888) (21.2436, 53.8162) (20.9564, 53.7311) knots 0 0 0 1 2 2 2
  line L30 (22.3845, 52.9785) -> (21.6186, 52.9785)
  spline S139 degree 2 poles (21.6186, 52.9785) (21.6159, 52.9386) (21.6159, 52.912) knots 0 0 0 1 1 1